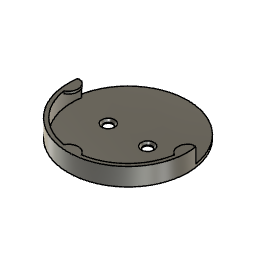
45mm Coin Holder (Autodesk Fusion 360 design; units mm, degrees)
Autodesk Fusion 360 part; units mm, degrees
note: some values were not read from the file. Set by a fixed rule: which face or edge a step refers to.
cylinder "CylinderPrimitive1" add diameter 44.5 height 4.5 placed x (1, 0, 0) y (0, 1, 0) z (0, 0, 1) at (0, 0, 0) makes body 1 in component "Coin"
sketch "Base" plane through (0, 0, 0) normal (0, 0, 1) x (1, 0, 0) in component "Coin Holder"
  circle A0 centre (0, 0) radius 22.25 construction
  circle A1 centre (0, 0) radius 22.75
  circle A2 centre (0, 0) radius 24.25
  dimension "d3" = 0.5
  dimension "d4" = 2
extrude "Extrude1" add sketch "Base" against normal blind 1.2 separate body contours A1 | A2 makes body 2 in component "Coin Holder"
extrude "Extrude2" add sketch "Base" along normal blind 5 bodies 2 in component "Coin Holder"
sketch "Holder Ears" plane through (0, 0, 5) normal (0, 0, 1) x (-1, 0, 0) in component "Coin Holder"
  circle A0 centre (0, 0) radius 22.75
  circle A1 centre (0, 0) radius 24.25
  line L0 (0, 0) -> (0, 24.25) construction
  arc A2 (-4, 24.2385) -> (3.9864, 23.9201) centre (0, 24.25) ccw
  dimension "d9" = 4
  constraint coincident A0.centre A1.centre
  constraint coincident A1 L0.end
  constraint vertical L0
  constraint coincident A1 A2.end
  constraint coincident L0.end A2.centre
  measures "d9" radius of A2
extrude "Extrude3" add sketch "Holder Ears" along normal blind 1 contours A0 A2 | A0 A1 A2 picked at (0.0985, 21.8993) picked at (-0.3993, 23.715) bodies 2 in component "Coin Holder"
pattern_circular "C-Pattern1" count 4 over 360 about axis through (0, 0, 1.75) along (0, 0, 1) of "Extrude3" in component "Coin Holder"
extrude "Extrude4" add 4 faces at (9.0692, -21.8969, 5) (21.8969, 9.0692, 5) (-9.0692, 21.8969, 5) (-21.8969, -9.0692, 5) along direction (0, 0, 1) blind 1 on bodies 2 bodies 2 in component "Coin Holder"
sketch "Mounting Holes" plane through (0, 0, 0) normal (0, 0, 1) x (1, 0, 0) in component "Coin Holder"
  line L0 (0, 0) -> (-8, 0) construction
  circle A0 centre (-8, 0) radius 2.55
  line L1 (0, 2.5) -> (0, 20)
  line L2 (0, 0) -> (8, 0) construction
  circle A1 centre (8, 0) radius 2.55
  point P0 (8, 0)
  dimension "d16" = 5.1
  dimension "d17" = 16
  constraint coincident L0.start L2.start
  constraint horizontal L0
  constraint coincident L0.end A0.centre
  constraint symmetric L0.start L1 L2.start
  constraint symmetric L0.end L1 P0
  constraint coincident P0 L2.end
  constraint equal A0 A1
  measures "d16" diameter of A0
  measures "d17" distance of L0.end P0
hole "Hole1" at (-8, 0, 0) at (8, 0, 0) direction (0, 0, -1) diameter 3.6 depth 12 tip angle 118 countersink diameter 5.3 countersink angle 90 bodies 2 in component "Coin Holder"
sketch "Top Trimmed off" plane through (0, 0, 6) normal (0, 0, 1) x (-1, 0, 0) in component "Coin Holder"
  circle A0 centre (0, 0) radius 24.25
  arc A1 (22.4665, 3.5804) -> (3.5804, 22.4665) centre (0, 0) ccw
  arc A2 (22.4665, 3.5804) -> (22.4665, -3.5804) centre (24.25, 0) ccw
  arc A3 (3.5804, -22.4665) -> (22.4665, -3.5804) centre (0, 0) ccw
  arc A4 (3.5804, -22.4665) -> (-3.5804, -22.4665) centre (0, -24.25) ccw
  arc A5 (-22.4665, -3.5804) -> (-3.5804, -22.4665) centre (0, 0) ccw
  arc A6 (-22.4665, -3.5804) -> (-22.4665, 3.5804) centre (-24.25, 0) ccw
  arc A7 (-3.5804, 22.4665) -> (-22.4665, 3.5804) centre (0, 0) ccw
  arc A8 (-3.5804, 22.4665) -> (3.5804, 22.4665) centre (0, 24.25) ccw
  line L0 (23.9842, -3.5804) -> (-22.4665, -3.5804)
  line L1 (-22.4665, -3.5804) -> (-23.9842, -3.5804)
  constraint coincident A0 L0.start
  constraint coincident A5.start A6.start
  constraint horizontal L0
  constraint coincident A0 L1.end
  constraint parallel L0 L1
extrude "Extrude5" cut sketch "Top Trimmed off" against normal blind 6 contours A0 A3 A4 A5 L0 L1 | A3 A4 A5 L0 bodies 2 in component "Coin Holder"
component "Coin" placed x (1, 0, 0) y (0, 1, 0) z (0, 0, 1) at (0, 0, 0)
component "Coin Holder" placed x (1, 0, 0) y (0, 1, 0) z (0, 0, 1) at (0, 0, 0)
named bodies: "Coin Model", "Coin Holder"
